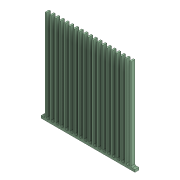
# Autodesk Inventor part: SGB-3-bins
Saved by Autodesk Inventor 2020 (Build 240168000, 168)
## iProperties
Created: 2021-06-24
Part Number: SGB-3-bins
Material: Generic
Document SubType Name: Modeling
Designer: Aidan Lee
Density: 1 g/cm^3
Appearance: Rubber - Green
Author: Aidan Lee
Autodesk Inventor part; units mm, degrees
ref_plane "YZ Plane" through (0, 0, 0) normal (1, 0, 0) x (0, 1, 0)
ref_plane "XZ Plane" through (0, 0, 0) normal (0, 1, 0) x (-1, 0, 0)
ref_plane "XY Plane" through (0, 0, 0) normal (0, 0, 1) x (1, 0, 0)
sketch "Sketch1" plane through (0, 0, 0) normal (0, 0, 1) x (1, 0, 0)
  line L0 (0, 0) -> (140, 0)
  line L1 (140, 0) -> (140, 300)
  line L2 (140, 300) -> (0, 300)
  line L3 (0, 300) -> (0, 0)
  line L4 (10, 290) -> (130, 290)
  line L5 (130, 290) -> (130, 10) construction
  line L6 (130, 10) -> (10, 10) construction
  line L7 (10, 10) -> (10, 290) construction
  line L8 (55.013, 210.0189) -> (44.1329, 210.0189) construction
  line L9 (10, 290) -> (130, 290) construction
  line L10 (70, 311.1686) -> (70, 319.6965) construction
  line L11 (64.8975, 210.0189) -> (64.8975, 204.1374) construction
  line L12 (75.1025, 210.0189) -> (75.1025, 204.1374) construction
  spline S0 degree 4 poles (64.8975, 210.0189) (64.8975, 218.5538) (47.6053, 225.9043) (40.8111, 229.8746) (18.3339, 245.7556) (11.7937, 258.2232) (10, 279.3922) (10, 290) knots 0 0 0 0 0 0.284812 0.471394 0.66948 1 1 1 1 1
  line L13 (10, 290) -> (10, 266.9306) construction
  spline S1 degree 4 poles (75.1025, 210.0189) (75.1025, 218.5538) (92.3947, 225.9043) (99.1889, 229.8746) (121.6661, 245.7556) (128.2063, 258.2232) (130, 279.3922) (130, 290) knots 0 0 0 0 0 0.284812 0.471394 0.66948 1 1 1 1 1
  spline S2 degree 4 poles (64.8975, 210.0189) (64.8975, 201.4839) (47.6053, 194.1334) (40.8111, 190.1632) (18.3339, 174.2821) (11.7937, 161.8145) (10, 140.6455) (10, 130.0377) knots 0 0 0 0 0 0.284812 0.471394 0.66948 1 1 1 1 1
  spline S3 degree 4 poles (75.1025, 210.0189) (75.1025, 201.4839) (92.3947, 194.1334) (99.1889, 190.1632) (121.6661, 174.2821) (128.2063, 161.8145) (130, 140.6455) (130, 130.0377) knots 0 0 0 0 0 0.284812 0.471394 0.66948 1 1 1 1 1
  line L14 (10, 130.0377) -> (10, 10)
  line L15 (130, 130.0377) -> (130, 10)
  line L16 (10, 10) -> (130, 10)
  line L17 (240, 186.8124) -> (240, 163.5372) construction
  line L18 (480, 0) -> (340, 0) construction
  line L19 (340, 0) -> (340, 300) construction
  line L20 (340, 300) -> (480, 300) construction
  line L21 (480, 300) -> (480, 0) construction
  line L22 (470, 290) -> (350, 290) construction
  line L23 (350, 290) -> (350, 10) construction
  line L24 (350, 10) -> (470, 10) construction
  line L25 (470, 10) -> (470, 290) construction
  line L26 (424.987, 210.0189) -> (435.8671, 210.0189) construction
  line L27 (470, 290) -> (350, 290) construction
  line L28 (410, 311.1686) -> (410, 319.6965) construction
  line L29 (415.1025, 210.0189) -> (415.1025, 204.1374) construction
  line L30 (404.8975, 210.0189) -> (404.8975, 204.1374) construction
  spline S4 degree 4 poles (415.1025, 210.0189) (415.1025, 218.5538) (432.3947, 225.9043) (439.1889, 229.8746) (461.6661, 245.7556) (468.2063, 258.2232) (470, 279.3922) (470, 290) knots 0 0 0 0 0 0.284812 0.471394 0.66948 1 1 1 1 1 construction
  line L31 (470, 290) -> (470, 266.9306) construction
  spline S5 degree 4 poles (404.8975, 210.0189) (394.814, 224.8509) (381.6315, 227.4313) (352.9317, 245.1456) (350.4567, 267.2032) (350, 290) knots 0 0 0 0 0 0.471394 1 1 1 1 1 construction
  spline S6 degree 4 poles (415.1025, 210.0189) (425.186, 195.1868) (438.3685, 192.6065) (467.0683, 174.8921) (469.5433, 152.8345) (470, 130.0377) knots 0 0 0 0 0 0.471394 1 1 1 1 1 construction
  spline S7 degree 4 poles (404.8975, 210.0189) (394.814, 195.1868) (381.6315, 192.6065) (352.9317, 174.8921) (350.4567, 152.8345) (350, 130.0377) knots 0 0 0 0 0 0.471394 1 1 1 1 1 construction
  line L32 (355, 14.5) -> (355, 130.0377)
  line L33 (355, 130.0377) -> (357, 130.0377)
  line L34 (357, 130.0377) -> (357, 14.5)
  arc A0 (353.5, 13) -> (355, 14.5) centre (353.5, 14.5) ccw
  arc A1 (351, 14.5) -> (352.5, 13) centre (352.5, 14.5) ccw construction
  line L35 (352.5, 13) -> (353.5, 13)
  arc A2 (357, 14.5) -> (358.5, 13) centre (358.5, 14.5) ccw
  line L36 (358.5, 13) -> (359.5, 13)
  line L37 (361, 14.5) -> (361, 130.0377)
  line L38 (363, 130.0377) -> (363, 14.5)
  arc A3 (359.5, 13) -> (361, 14.5) centre (359.5, 14.5) ccw
  line L39 (361, 130.0377) -> (363, 130.0377)
  arc A4 (363, 14.5) -> (364.5, 13) centre (364.5, 14.5) ccw
  line L40 (364.5, 13) -> (365.5, 13)
  line L41 (367, 14.5) -> (367, 130.0377)
  line L42 (369, 130.0377) -> (369, 14.5)
  arc A5 (365.5, 13) -> (367, 14.5) centre (365.5, 14.5) ccw
  line L43 (367, 130.0377) -> (369, 130.0377)
  arc A6 (369, 14.5) -> (370.5, 13) centre (370.5, 14.5) ccw
  line L44 (370.5, 13) -> (371.5, 13)
  line L45 (373, 14.5) -> (373, 130.0377)
  line L46 (375, 130.0377) -> (375, 14.5)
  arc A7 (371.5, 13) -> (373, 14.5) centre (371.5, 14.5) ccw
  line L47 (373, 130.0377) -> (375, 130.0377)
  arc A8 (375, 14.5) -> (376.5, 13) centre (376.5, 14.5) ccw
  line L48 (376.5, 13) -> (377.5, 13)
  line L49 (379, 14.5) -> (379, 130.0377)
  line L50 (381, 130.0377) -> (381, 14.5)
  arc A9 (377.5, 13) -> (379, 14.5) centre (377.5, 14.5) ccw
  line L51 (379, 130.0377) -> (381, 130.0377)
  arc A10 (381, 14.5) -> (382.5, 13) centre (382.5, 14.5) ccw
  line L52 (382.5, 13) -> (383.5, 13)
  line L53 (385, 14.5) -> (385, 130.0377)
  line L54 (387, 130.0377) -> (387, 14.5)
  arc A11 (383.5, 13) -> (385, 14.5) centre (383.5, 14.5) ccw
  line L55 (385, 130.0377) -> (387, 130.0377)
  arc A12 (387, 14.5) -> (388.5, 13) centre (388.5, 14.5) ccw
  line L56 (388.5, 13) -> (389.5, 13)
  line L57 (391, 14.5) -> (391, 130.0377)
  line L58 (393, 130.0377) -> (393, 14.5)
  arc A13 (389.5, 13) -> (391, 14.5) centre (389.5, 14.5) ccw
  line L59 (391, 130.0377) -> (393, 130.0377)
  arc A14 (393, 14.5) -> (394.5, 13) centre (394.5, 14.5) ccw
  line L60 (394.5, 13) -> (395.5, 13)
  line L61 (397, 14.5) -> (397, 130.0377)
  line L62 (399, 130.0377) -> (399, 14.5)
  arc A15 (395.5, 13) -> (397, 14.5) centre (395.5, 14.5) ccw
  line L63 (397, 130.0377) -> (399, 130.0377)
  arc A16 (399, 14.5) -> (400.5, 13) centre (400.5, 14.5) ccw
  line L64 (400.5, 13) -> (401.5, 13)
  line L65 (403, 14.5) -> (403, 130.0377)
  line L66 (405, 130.0377) -> (405, 14.5)
  arc A17 (401.5, 13) -> (403, 14.5) centre (401.5, 14.5) ccw
  line L67 (403, 130.0377) -> (405, 130.0377)
  arc A18 (405, 14.5) -> (406.5, 13) centre (406.5, 14.5) ccw
  line L68 (406.5, 13) -> (407.5, 13)
  line L69 (409, 14.5) -> (409, 130.0377)
  line L70 (411, 130.0377) -> (411, 14.5)
  arc A19 (407.5, 13) -> (409, 14.5) centre (407.5, 14.5) ccw
  line L71 (409, 130.0377) -> (411, 130.0377)
  arc A20 (411, 14.5) -> (412.5, 13) centre (412.5, 14.5) ccw
  line L72 (412.5, 13) -> (413.5, 13)
  line L73 (415, 14.5) -> (415, 130.0377)
  line L74 (417, 130.0377) -> (417, 14.5)
  arc A21 (413.5, 13) -> (415, 14.5) centre (413.5, 14.5) ccw
  line L75 (415, 130.0377) -> (417, 130.0377)
  arc A22 (417, 14.5) -> (418.5, 13) centre (418.5, 14.5) ccw
  line L76 (418.5, 13) -> (419.5, 13)
  line L77 (421, 14.5) -> (421, 130.0377)
  line L78 (423, 130.0377) -> (423, 14.5)
  arc A23 (419.5, 13) -> (421, 14.5) centre (419.5, 14.5) ccw
  line L79 (421, 130.0377) -> (423, 130.0377)
  arc A24 (423, 14.5) -> (424.5, 13) centre (424.5, 14.5) ccw
  line L80 (424.5, 13) -> (425.5, 13)
  line L81 (427, 14.5) -> (427, 130.0377)
  line L82 (429, 130.0377) -> (429, 14.5)
  arc A25 (425.5, 13) -> (427, 14.5) centre (425.5, 14.5) ccw
  line L83 (427, 130.0377) -> (429, 130.0377)
  arc A26 (429, 14.5) -> (430.5, 13) centre (430.5, 14.5) ccw
  line L84 (430.5, 13) -> (431.5, 13)
  line L85 (433, 14.5) -> (433, 130.0377)
  line L86 (435, 130.0377) -> (435, 14.5)
  arc A27 (431.5, 13) -> (433, 14.5) centre (431.5, 14.5) ccw
  line L87 (433, 130.0377) -> (435, 130.0377)
  arc A28 (435, 14.5) -> (436.5, 13) centre (436.5, 14.5) ccw
  line L88 (436.5, 13) -> (437.5, 13)
  line L89 (439, 14.5) -> (439, 130.0377)
  line L90 (441, 130.0377) -> (441, 14.5)
  arc A29 (437.5, 13) -> (439, 14.5) centre (437.5, 14.5) ccw
  line L91 (439, 130.0377) -> (441, 130.0377)
  arc A30 (441, 14.5) -> (442.5, 13) centre (442.5, 14.5) ccw
  line L92 (442.5, 13) -> (443.5, 13)
  line L93 (445, 14.5) -> (445, 130.0377)
  line L94 (447, 130.0377) -> (447, 14.5)
  arc A31 (443.5, 13) -> (445, 14.5) centre (443.5, 14.5) ccw
  line L95 (445, 130.0377) -> (447, 130.0377)
  arc A32 (447, 14.5) -> (448.5, 13) centre (448.5, 14.5) ccw
  line L96 (448.5, 13) -> (449.5, 13)
  line L97 (451, 14.5) -> (451, 130.0377)
  line L98 (453, 130.0377) -> (453, 14.5)
  arc A33 (449.5, 13) -> (451, 14.5) centre (449.5, 14.5) ccw
  line L99 (451, 130.0377) -> (453, 130.0377)
  arc A34 (453, 14.5) -> (454.5, 13) centre (454.5, 14.5) ccw
  line L100 (454.5, 13) -> (455.5, 13)
  line L101 (457, 14.5) -> (457, 130.0377)
  line L102 (459, 130.0377) -> (459, 14.5)
  arc A35 (455.5, 13) -> (457, 14.5) centre (455.5, 14.5) ccw
  line L103 (457, 130.0377) -> (459, 130.0377)
  arc A36 (459, 14.5) -> (460.5, 13) centre (460.5, 14.5) ccw
  line L104 (460.5, 13) -> (461.5, 13)
  line L105 (463, 14.5) -> (463, 130.0377)
  line L106 (465, 130.0377) -> (465, 14.5)
  arc A37 (461.5, 13) -> (463, 14.5) centre (461.5, 14.5) ccw
  line L107 (463, 130.0377) -> (465, 130.0377)
  arc A38 (465, 14.5) -> (466.5, 13) centre (466.5, 14.5) ccw
  line L108 (466.5, 13) -> (470, 13)
  line L109 (470, 10) -> (470, 13)
  line L110 (470, 10) -> (350, 10)
  line L111 (350, 10) -> (350, 13)
  line L112 (352.5, 13) -> (350, 13)
  line L113 (740, 300) -> (600, 300)
  line L114 (610, 290) -> (730, 290) construction
  line L115 (610, 290) -> (730, 290) construction
  spline S8 degree 4 poles (675.1025, 210.0189) (675.1025, 218.5538) (692.3947, 225.9043) (699.1889, 229.8746) (721.6661, 245.7556) (728.2063, 258.2232) (730, 279.3922) (730, 290) knots 0 0 0 0 0 0.284812 0.471394 0.66948 1 1 1 1 1 construction
  line L116 (664.8975, 210.0189) -> (664.8975, 204.1374) construction
  line L117 (610, 290) -> (610, 266.9306) construction
  spline S9 degree 4 poles (664.8975, 210.0189) (664.8975, 218.5538) (647.6053, 225.9043) (640.8111, 229.8746) (618.3339, 245.7556) (611.7937, 258.2232) (610, 279.3922) (610, 290) knots 0 0 0 0 0 0.284812 0.471394 0.66948 1 1 1 1 1 construction
  line L118 (675.1025, 210.0189) -> (675.1025, 204.1374) construction
  spline S10 degree 4 poles (675.1025, 210.0189) (675.1025, 201.4839) (692.3947, 194.1334) (699.1889, 190.1632) (721.6661, 174.2821) (728.2063, 161.8145) (730, 140.6455) (730, 130.0377) knots 0 0 0 0 0 0.284812 0.471394 0.66948 1 1 1 1 1 construction
  spline S11 degree 4 poles (664.8975, 210.0189) (664.8975, 201.4839) (647.6053, 194.1334) (640.8111, 190.1632) (618.3339, 174.2821) (611.7937, 161.8145) (610, 140.6455) (610, 130.0377) knots 0 0 0 0 0 0.284812 0.471394 0.66948 1 1 1 1 1 construction
  line L119 (730, 290) -> (730, 10) construction
  line L120 (610, 10) -> (610, 290) construction
  line L121 (740, 0) -> (740, 300)
  line L122 (600, 300) -> (600, 0)
  line L123 (610, 130.0377) -> (610, 10) construction
  line L124 (730, 10) -> (610, 10) construction
  line L125 (610, 10) -> (730, 10) construction
  line L126 (730, 130.0377) -> (730, 10) construction
  line L127 (600, 0) -> (740, 0)
  circle A39 centre (670, 187.6403) radius 1.45
  line L128 (661.5147, 179.155) -> (670, 187.6403) construction
  line L129 (670, 187.6403) -> (661.5147, 179.155) construction
  line L130 (661.5147, 179.155) -> (678.4853, 179.155) construction
  line L131 (130, 290) -> (130, 293.3347) construction
  line L132 (730, 290) -> (730, 294.5645) construction
  line L133 (670, 187.6403) -> (667.2579, 190.3824) construction
  line L134 (661.5147, 179.155) -> (658.7726, 181.8971) construction
  circle A40 centre (661.5147, 179.155) radius 1.45
  circle A41 centre (653.0294, 170.6697) radius 1.45
  circle A42 centre (644.5442, 162.1844) radius 1.45
  circle A43 centre (636.0589, 153.6991) radius 1.45
  circle A44 centre (627.5736, 145.2139) radius 1.45
  circle A45 centre (619.0883, 136.7286) radius 1.45
  circle A46 centre (619.0883, 153.6991) radius 1.45
  circle A47 centre (627.5736, 162.1844) radius 1.45
  circle A48 centre (636.0589, 170.6697) radius 1.45
  circle A49 centre (644.5442, 179.155) radius 1.45
  circle A50 centre (653.0294, 187.6403) radius 1.45
  circle A51 centre (686.9706, 187.6403) radius 1.45
  circle A52 centre (678.4853, 179.155) radius 1.45
  circle A53 centre (670, 170.6697) radius 1.45
  circle A54 centre (661.5147, 162.1844) radius 1.45
  circle A55 centre (653.0294, 153.6991) radius 1.45
  circle A56 centre (644.5442, 145.2139) radius 1.45
  circle A57 centre (636.0589, 136.7286) radius 1.45
  circle A58 centre (695.4558, 179.155) radius 1.45
  circle A59 centre (686.9706, 170.6697) radius 1.45
  circle A60 centre (670, 170.6697) radius 1.45
  circle A61 centre (661.5147, 162.1844) radius 1.45
  circle A62 centre (678.4853, 162.1844) radius 1.45
  circle A63 centre (653.0294, 153.6991) radius 1.45
  circle A64 centre (670, 153.6991) radius 1.45
  circle A65 centre (661.5147, 145.2139) radius 1.45
  circle A66 centre (644.5442, 145.2139) radius 1.45
  circle A67 centre (636.0589, 136.7286) radius 1.45
  circle A68 centre (653.0294, 136.7286) radius 1.45
  circle A69 centre (695.4558, 162.1844) radius 1.45
  circle A70 centre (686.9706, 153.6991) radius 1.45
  circle A71 centre (678.4853, 145.2139) radius 1.45
  circle A72 centre (670, 136.7286) radius 1.45
  circle A73 centre (712.4264, 162.1844) radius 1.45
  circle A74 centre (703.9411, 153.6991) radius 1.45
  circle A75 centre (695.4558, 145.2139) radius 1.45
  circle A76 centre (686.9706, 136.7286) radius 1.45
  circle A77 centre (703.9411, 170.6697) radius 1.45
  circle A78 centre (720.9117, 153.6991) radius 1.45
  circle A79 centre (712.4264, 145.2139) radius 1.45
  circle A80 centre (703.9411, 136.7286) radius 1.45
  circle A81 centre (720.9117, 136.7286) radius 1.45
  line L135 (0, 160.5) -> (-18, 160.5)
  line L136 (-18, 160.5) -> (-18, 180.5)
  line L137 (-18, 180.5) -> (0, 180.5) construction
  line L138 (0, 180.5) -> (0, 160.5)
  line L139 (-24.3067, 150) -> (-34.4998, 150) construction
  circle A82 centre (-9, 170.5) radius 3
  line L140 (-18, 180.5) -> (0, 200.5)
  line L141 (0, 139.5) -> (-18, 139.5)
  line L142 (-18, 139.5) -> (-18, 119.5)
  circle A83 centre (-9, 129.5) radius 3
  line L143 (-18, 119.5) -> (0, 99.5)
  line L144 (140, 160.5) -> (158, 160.5)
  line L145 (158, 160.5) -> (158, 180.5)
  circle A84 centre (149, 170.5) radius 3
  line L146 (158, 180.5) -> (140, 200.5)
  line L147 (158, 139.5) -> (158, 119.5)
  line L148 (140, 139.5) -> (158, 139.5)
  circle A85 centre (149, 129.5) radius 3
  line L149 (158, 119.5) -> (140, 99.5)
  line L150 (582, 180.5) -> (600, 200.5)
  line L151 (582, 160.5) -> (582, 180.5)
  circle A86 centre (591, 170.5) radius 3
  line L152 (600, 139.5) -> (582, 139.5)
  circle A87 centre (591, 129.5) radius 3
  line L153 (582, 139.5) -> (582, 119.5)
  line L154 (582, 119.5) -> (600, 99.5)
  line L155 (758, 180.5) -> (740, 200.5)
  line L156 (758, 160.5) -> (758, 180.5)
  circle A88 centre (749, 170.5) radius 3
  line L157 (740, 160.5) -> (758, 160.5)
  line L158 (740, 139.5) -> (758, 139.5)
  circle A89 centre (749, 129.5) radius 3
  line L159 (758, 139.5) -> (758, 119.5)
  line L160 (758, 119.5) -> (740, 99.5)
  line L161 (600, 160.5) -> (582, 160.5)
  line L162 (600, 200.5) -> (600, 300)
  line L163 (600, 300) -> (740, 300)
  line L164 (740, 300) -> (740, 200.5)
  line L165 (740, 160.5) -> (740, 139.5)
  line L166 (740, 99.5) -> (740, 0)
  line L167 (740, 0) -> (600, 0)
  line L168 (600, 0) -> (600, 99.5)
  line L169 (600, 139.5) -> (600, 160.5)
  line L170 (780, 153.6991) -> (780, 161.6118) construction
  line L171 (820, 300) -> (960, 300)
  line L172 (960, 0) -> (820, 0)
  line L173 (978, 180.5) -> (960, 200.5)
  line L174 (978, 160.5) -> (978, 180.5)
  circle A90 centre (969, 170.5) radius 3
  line L175 (960, 139.5) -> (978, 139.5)
  circle A91 centre (969, 129.5) radius 3
  line L176 (978, 139.5) -> (978, 119.5)
  line L177 (978, 119.5) -> (960, 99.5)
  line L178 (802, 180.5) -> (820, 200.5)
  line L179 (802, 160.5) -> (802, 180.5)
  circle A92 centre (811, 170.5) radius 3
  line L180 (820, 160.5) -> (802, 160.5)
  line L181 (820, 139.5) -> (802, 139.5)
  circle A93 centre (811, 129.5) radius 3
  line L182 (802, 139.5) -> (802, 119.5)
  line L183 (802, 119.5) -> (820, 99.5)
  line L184 (960, 160.5) -> (978, 160.5)
  line L185 (960, 200.5) -> (960, 300)
  line L186 (960, 300) -> (820, 300)
  line L187 (820, 300) -> (820, 200.5)
  line L188 (820, 160.5) -> (820, 139.5)
  line L189 (820, 99.5) -> (820, 0)
  line L190 (820, 0) -> (960, 0)
  line L191 (960, 0) -> (960, 99.5)
  line L192 (960, 139.5) -> (960, 160.5)
  line L193 (582, -180.5) -> (582, -200.5) construction
  circle A94 centre (591, -190.5) radius 3 construction
  line L194 (600, -159.5) -> (582, -159.5) construction
  line L195 (600, -180.5) -> (582, -180.5) construction
  line L196 (582, -200.5) -> (600, -220.5) construction
  line L197 (582, -139.5) -> (600, -119.5) construction
  line L198 (582, -159.5) -> (582, -139.5) construction
  circle A95 centre (591, -149.5) radius 3 construction
  circle A96 centre (619.0883, -166.3009) radius 1.45 construction
  circle A97 centre (627.5736, -174.7861) radius 1.45 construction
  circle A98 centre (644.5442, -157.8156) radius 1.45 construction
  circle A99 centre (627.5736, -157.8156) radius 1.45 construction
  circle A100 centre (644.5442, -174.7861) radius 1.45 construction
  circle A101 centre (636.0589, -183.2714) radius 1.45 construction
  line L199 (600, -180.5) -> (600, -159.5) construction
  circle A102 centre (636.0589, -183.2714) radius 1.45 construction
  circle A103 centre (644.5442, -174.7861) radius 1.45 construction
  circle A104 centre (619.0883, -183.2714) radius 1.45 construction
  circle A105 centre (636.0589, -166.3009) radius 1.45 construction
  circle A106 centre (653.0294, -183.2714) radius 1.45 construction
  circle A107 centre (661.5147, -174.7861) radius 1.45 construction
  line L200 (664.8975, -109.9811) -> (664.8975, -115.8626) construction
  line L201 (610, -30) -> (610, -53.0694) construction
  spline S12 degree 4 poles (664.8975, -109.9811) (664.8975, -118.5161) (647.6053, -125.8666) (640.8111, -129.8368) (618.3339, -145.7179) (611.7937, -158.1855) (610, -179.3545) (610, -189.9623) knots 0 0 0 0 0 0.284812 0.471394 0.66948 1 1 1 1 1 construction
  circle A108 centre (670, -149.3303) radius 1.45 construction
  circle A109 centre (678.4853, -140.845) radius 1.45 construction
  circle A110 centre (686.9706, -166.3009) radius 1.45 construction
  circle A111 centre (670, -166.3009) radius 1.45 construction
  circle A112 centre (653.0294, -166.3009) radius 1.45 construction
  circle A113 centre (653.0294, -166.3009) radius 1.45 construction
  spline S13 degree 4 poles (664.8975, -109.9811) (664.8975, -101.4462) (647.6053, -94.0957) (640.8111, -90.1254) (618.3339, -74.2444) (611.7937, -61.7768) (610, -40.6078) (610, -30) knots 0 0 0 0 0 0.284812 0.471394 0.66948 1 1 1 1 1 construction
  circle A114 centre (670, -132.3597) radius 1.45 construction
  circle A115 centre (636.0589, -149.3303) radius 1.45 construction
  circle A116 centre (653.0294, -149.3303) radius 1.45 construction
  circle A117 centre (644.5442, -140.845) radius 1.45 construction
  circle A118 centre (653.0294, -132.3597) radius 1.45 construction
  line L202 (661.5147, -140.845) -> (658.7726, -138.1029) construction
  line L203 (661.5147, -140.845) -> (670, -132.3597) construction
  line L204 (670, -132.3597) -> (661.5147, -140.845) construction
  line L205 (670, -132.3597) -> (667.2579, -129.6176) construction
  line L206 (661.5147, -140.845) -> (678.4853, -140.845) construction
  circle A119 centre (686.9706, -132.3597) radius 1.45 construction
  line L207 (600, -119.5) -> (600, -20) construction
  line L208 (600, -20) -> (740, -20) construction
  line L209 (730, -30) -> (730, -25.4355) construction
  line L210 (740, -20) -> (740, -119.5) construction
  circle A120 centre (661.5147, -140.845) radius 1.45 construction
  line L211 (610, -189.9623) -> (610, -310) construction
  line L212 (600, -320) -> (600, -220.5) construction
  line L213 (730, -310) -> (610, -310) construction
  line L214 (610, -310) -> (730, -310) construction
  line L215 (600, -320) -> (740, -320) construction
  line L216 (740, -320) -> (600, -320) construction
  line L217 (730, -189.9623) -> (730, -310) construction
  line L218 (740, -220.5) -> (740, -320) construction
  line L219 (740, -20) -> (600, -20) construction
  line L220 (675.1025, -109.9811) -> (675.1025, -115.8626) construction
  line L221 (610, -30) -> (730, -30) construction
  line L222 (610, -30) -> (730, -30) construction
  spline S14 degree 4 poles (675.1025, -109.9811) (675.1025, -101.4462) (692.3947, -94.0957) (699.1889, -90.1254) (721.6661, -74.2444) (728.2063, -61.7768) (730, -40.6078) (730, -30) knots 0 0 0 0 0 0.284812 0.471394 0.66948 1 1 1 1 1 construction
  line L223 (610, -310) -> (610, -30) construction
  line L224 (600, -20) -> (600, -320) construction
  line L225 (740, -320) -> (740, -20) construction
  line L226 (730, -30) -> (730, -310) construction
  circle A121 centre (678.4853, -174.7861) radius 1.45 construction
  circle A122 centre (670, -183.2714) radius 1.45 construction
  spline S15 degree 4 poles (675.1025, -109.9811) (675.1025, -118.5161) (692.3947, -125.8666) (699.1889, -129.8368) (721.6661, -145.7179) (728.2063, -158.1855) (730, -179.3545) (730, -189.9623) knots 0 0 0 0 0 0.284812 0.471394 0.66948 1 1 1 1 1 construction
  circle A123 centre (686.9706, -183.2714) radius 1.45 construction
  circle A124 centre (670, -149.3303) radius 1.45 construction
  circle A125 centre (661.5147, -157.8156) radius 1.45 construction
  circle A126 centre (695.4558, -140.845) radius 1.45 construction
  circle A127 centre (686.9706, -149.3303) radius 1.45 construction
  circle A128 centre (678.4853, -157.8156) radius 1.45 construction
  circle A129 centre (703.9411, -149.3303) radius 1.45 construction
  line L227 (758, -139.5) -> (740, -119.5) construction
  circle A130 centre (749, -149.5) radius 3 construction
  line L228 (758, -159.5) -> (758, -139.5) construction
  circle A131 centre (661.5147, -157.8156) radius 1.45 construction
  circle A132 centre (703.9411, -183.2714) radius 1.45 construction
  circle A133 centre (712.4264, -174.7861) radius 1.45 construction
  circle A134 centre (720.9117, -183.2714) radius 1.45 construction
  circle A135 centre (695.4558, -174.7861) radius 1.45 construction
  line L229 (740, -159.5) -> (740, -180.5) construction
  line L230 (758, -200.5) -> (740, -220.5) construction
  circle A136 centre (749, -190.5) radius 3 construction
  line L231 (758, -180.5) -> (758, -200.5) construction
  line L232 (740, -180.5) -> (758, -180.5) construction
  line L233 (740, -159.5) -> (758, -159.5) construction
  circle A137 centre (720.9117, -166.3009) radius 1.45 construction
  circle A138 centre (703.9411, -166.3009) radius 1.45 construction
  circle A139 centre (695.4558, -157.8156) radius 1.45 construction
  circle A140 centre (712.4264, -157.8156) radius 1.45 construction
  line L234 (600, -122.3597) -> (740, -122.3597)
  line L235 (740, -122.3597) -> (740, -193.2714)
  line L236 (740, -193.2714) -> (600, -193.2714)
  line L237 (600, -193.2714) -> (600, -122.3597)
  point P0 (70, 290)
  point P1 (70, 300)
  point P2 (10, 150)
  point P3 (0, 150)
  point P4 (70, 290)
  point P5 (70, 315.4325)
  point P6 (49.5729, 210.0189)
  point P7 (49.5729, 225.4245)
  point P8 (37.5413, 232.3974)
  point P9 (24.0774, 242.8841)
  point P10 (14.2457, 257.8533)
  point P11 (90.4271, 225.4245)
  point P12 (102.4587, 232.3974)
  point P13 (115.9226, 242.8841)
  point P14 (125.7543, 257.8533)
  point P15 (49.5729, 194.6132)
  point P16 (37.5413, 187.6403)
  point P17 (24.0774, 177.1536)
  point P18 (14.2457, 162.1844)
  point P19 (90.4271, 194.6132)
  point P20 (102.4587, 187.6403)
  point P21 (115.9226, 177.1536)
  point P22 (125.7543, 162.1844)
  point P23 (410, 290)
  point P24 (410, 300)
  point P25 (470, 150)
  point P26 (480, 150)
  point P27 (410, 290)
  point P28 (410, 315.4325)
  point P29 (430.4271, 210.0189)
  point P30 (430.4271, 225.4245)
  point P31 (442.4587, 232.3974)
  point P32 (455.9226, 242.8841)
  point P33 (465.7543, 257.8533)
  point P34 (389.5729, 225.4245)
  point P35 (377.5413, 232.3974)
  point P36 (364.0774, 242.8841)
  point P37 (354.2457, 257.8533)
  point P38 (430.4271, 194.6132)
  point P39 (442.4587, 187.6403)
  point P40 (455.9226, 177.1536)
  point P41 (465.7543, 162.1844)
  point P42 (389.5729, 194.6132)
  point P43 (377.5413, 187.6403)
  point P44 (364.0774, 177.1536)
  point P45 (354.2457, 162.1844)
  point P46 (356, 130.0377)
  point P47 (362, 130.0377)
  point P48 (368, 130.0377)
  point P49 (374, 130.0377)
  point P50 (380, 130.0377)
  point P51 (386, 130.0377)
  point P52 (392, 130.0377)
  point P53 (398, 130.0377)
  point P54 (404, 130.0377)
  point P55 (410, 130.0377)
  point P56 (416, 130.0377)
  point P57 (422, 130.0377)
  point P58 (428, 130.0377)
  point P59 (434, 130.0377)
  point P60 (440, 130.0377)
  point P61 (446, 130.0377)
  point P62 (452, 130.0377)
  point P63 (458, 130.0377)
  point P64 (464, 130.0377)
  point P65 (410, 130.0377)
  point P66 (410, 315.4325)
  point P67 (670, 300)
  point P68 (670, 290)
  point P69 (670, 290)
  point P70 (690.4271, 225.4245)
  point P71 (702.4587, 232.3974)
  point P72 (715.9226, 242.8841)
  point P73 (725.7543, 257.8533)
  point P74 (649.5729, 225.4245)
  point P75 (637.5413, 232.3974)
  point P76 (624.0774, 242.8841)
  point P77 (614.2457, 257.8533)
  point P78 (690.4271, 194.6132)
  point P79 (649.5729, 194.6132)
  point P80 (702.4587, 187.6403)
  point P81 (637.5413, 187.6403)
  point P82 (715.9226, 177.1536)
  point P83 (624.0774, 177.1536)
  point P84 (614.2457, 162.1844)
  point P85 (725.7543, 162.1844)
  point P86 (610, 150)
  point P87 (600, 150)
  point P88 (670, 179.155)
  point P89 (670, 300)
  point P90 (-29.4032, 150)
  point P91 (-18, 170.5)
  point P92 (-9, 180.5)
  point P93 (582, 170.5)
  point P94 (890, 300)
  point P95 (960, 150)
  point P96 (890, 300)
  point P97 (978, 170.5)
  point P98 (582, -149.5)
  point P99 (600, -170)
  point P100 (670, -30)
  point P101 (670, -30)
  point P102 (670, -20)
  point P103 (637.5413, -132.3597)
  point P104 (624.0774, -142.8464)
  point P105 (614.2457, -157.8156)
  point P106 (649.5729, -125.3868)
  point P107 (610, -170)
  point P108 (670, -140.845)
  point P109 (649.5729, -94.5755)
  point P110 (637.5413, -87.6026)
  point P111 (624.0774, -77.1159)
  point P112 (614.2457, -62.1467)
  point P113 (670, -20)
  point P114 (690.4271, -94.5755)
  point P115 (702.4587, -87.6026)
  point P116 (725.7543, -62.1467)
  point P117 (702.4587, -132.3597)
  point P118 (715.9226, -77.1159)
  point P119 (690.4271, -125.3868)
  point P120 (715.9226, -142.8464)
  point P121 (725.7543, -157.8156)
  point P122 (459, 14.5)
  point P123 (453, 14.5)
  point P124 (447, 14.5)
  point P125 (441, 14.5)
  point P126 (435, 14.5)
  point P127 (429, 14.5)
  point P128 (423, 14.5)
  point P129 (417, 14.5)
  point P130 (411, 14.5)
  point P131 (399, 14.5)
  point P132 (393, 14.5)
  point P133 (381, 14.5)
  point P134 (363, 14.5)
  dimension "d0" = 140
  dimension "d1" = 300
  dimension "d2" = 10
  dimension "d3" = 10
  dimension "d5" = 100
  dimension "d6" = 2
  dimension "d9" = 79.9811
  dimension "d12" = 1.5
  dimension "d13" = 1.5
  dimension "d15" = 4
  dimension "d18" = 6
  dimension "d23" = 3
  dimension "d26" = 600
  dimension "d33" = 2.9
  dimension "d34" = 45
  dimension "d35" = 12
  dimension "d38" = 12
  dimension "d45" = 16.9706
  dimension "d52" = 16.9706
  dimension "d59" = 16.9706
  dimension "d66" = 16.9706
  dimension "d73" = 16.9706
  dimension "d80" = 16.9706
  dimension "d85" = 18
  dimension "d86" = 20
  dimension "d87" = 10.5
  dimension "d88" = 6
  dimension "d89" = 20
  dimension "d92" = 600
  dimension "d97" = 10.2051
  dimension "d98" = 40
  dimension "d101" = 320
  dimension "d106" = 10
  dimension "d107" = 10
  constraints: 476 end point, 141 centre point, 101 symmetric about line, 78 point on circle, 25 vertical, 23 horizontal, 19 horizontal alignment, 15 midpoint, 15 vertical alignment, 11 collinear, 9 parallel, 9 perpendicular, 7 point on line, 2 tangent, 1 coincident, 759 other
  measures "d0" distance of L0.start L0.end
  measures "d1" distance of L2.end L0.start
  measures "d2" distance between parallel lines of L2 L4
  measures "d3" distance between parallel lines of L3 L7
  measures "d5" distance between parallel lines of L1 L17
  measures "d6" distance of L32.end L33.end
  measures "d9" vertical distance of point (49.573, 210.019) L14.start
  measures "d12" radius of A0
  measures "d13" radius of A1
  measures "d15" distance of L32.start A1.start
  measures "d18" distance of A1.centre A2.centre
  measures "d23" distance between parallel lines of L24 L35
  measures "d26" distance of L1.end L113.start
  measures "d33" diameter of A39
  measures "d34" angle of L130 L129
  measures "d35" distance between parallel lines of L133 L134
  measures "d38" distance of L128.end A40.centre
  measures "d45" distance of A43.centre A46.centre
  measures "d52" distance of L128.end A51.centre
  measures "d59" distance of A52.centre A58.centre
  measures "d66" distance of A62.centre A69.centre
  measures "d73" distance of A59.centre A77.centre
  measures "d80" distance of A76.centre A80.centre
  measures "d85" distance of L136.end L137.end
  measures "d86" distance of L135.end L136.end
  measures "d87" distance between parallel lines of L135 L139
  measures "d88" diameter of A82
  measures "d89" vertical distance of L136.end L140.end
  measures "d92" distance of L136.end L150.start
  measures "d97" distance between parallel lines of L12 L11
  measures "d98" distance from line of L113.start L170
  measures "d101" distance of L114.start L201.start
  measures "d106" distance from line of L234 A118.centre
  measures "d107" distance from line of L236 A104.centre
extrude "Extrusion1" add sketch "Sketch1" along normal blind 5 contours L32 L33 L34 A2 L36 A3 L37 L39 L38 A4 L40 A5 L41 L43 L42 A6 L44 A7 L45 L47 L46 A8 L48 A9 L49 L51 L50 A10 L52 A11 L53 L55 L54 A12 L56 A13 L57 L59 L58 A14 L60 A15 L61 L63 L62 A16 L64 A17 L65 L67 L66 A18 L68 A19 L69 L71 L70 A20 L72 A21 L73 L75 L74 A22 L76 A23 L77 L79 L78 A24 L80 A25 L81 L83 L82 A26 L84 A27 L85 L87 L86 A28 L88 A29 L89 L91 L90 A30 L92 A31 L93 L95 L94 A32 L96 A33 L97 L99 L98 A34 L100 A35 L101 L103 L102 A36 L104 A37 L105 L107 L106 A38 L108 L109 L110 L111 L112 L35 A0
body "Solid1"
